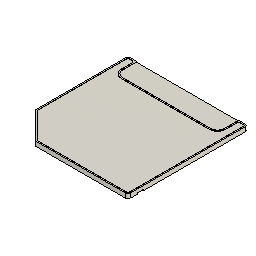
L_Floppy_Disk_v4 (Autodesk Fusion 360 design; units mm, degrees)
Autodesk Fusion 360 part; units mm, degrees
sketch "Sketch1" plane through (0, 0, 0) normal (0, 0, 1) x (1, 0, 0)
  line L0 (-64, 66.5) -> (64, 66.5)
  line L1 (66.5, 64) -> (66.5, -64)
  line L2 (64, -66.5) -> (-36.5, -66.5)
  line L3 (-66.5, -36.5) -> (-66.5, 64)
  line L4 (-36.5, -66.5) -> (-66.5, -36.5)
  arc A0 (-64, 66.5) -> (-66.5, 64) centre (-64, 64) ccw
  arc A1 (66.5, 64) -> (64, 66.5) centre (64, 64) ccw
  arc A2 (64, -66.5) -> (66.5, -64) centre (64, -64) ccw
extrude "Extrude1" add sketch "Sketch1" along normal blind 5
sketch "Sketch2" plane through (0, 0, 5) normal (0, 0, 1) x (-1, 0, 0)
  line L0 (36.5, 66.5) -> (-64, 66.5)
  arc A0 (-64, 66.5) -> (-66.5, 64) centre (-64, 64) ccw
  line L1 (-66.5, 64) -> (-66.5, -64)
  arc A1 (-66.5, -64) -> (-64, -66.5) centre (-64, -64) ccw
  line L2 (-64, -66.5) -> (64, -66.5)
  arc A2 (64, -66.5) -> (66.5, -64) centre (64, -64) ccw
  line L3 (66.5, -64) -> (66.5, 36.5)
  line L4 (66.5, 36.5) -> (36.5, 66.5)
  circle A3 centre (0, 0) radius 20
  circle A4 centre (0, 0) radius 16.5
  line L5 (-56.5, -66.5) -> (56.5, -66.5)
  line L6 (56.5, -66.5) -> (56.5, -50.5727)
  line L7 (49, -43.0727) -> (-49, -43.0727)
  line L8 (-56.5, -50.5727) -> (-56.5, -66.5)
  arc A5 (56.5, -50.5727) -> (49, -43.0727) centre (49, -50.5727) ccw
  arc A6 (-49, -43.0727) -> (-56.5, -50.5727) centre (-49, -50.5727) ccw
  constraint coincident A3.centre A4.centre
  constraint horizontal L5
  constraint equal A5 A6
extrude "Extrude2" cut sketch "Sketch2" against normal blind 0.2 contours L2 L5 L6 L7 L8 A5 A6
extrude "Extrude3" cut 1 faces at (16.3333, 58.6909, 4.8) along direction (0, 0, 1) blind 0.2 from surface at -4.8
sketch "Sketch3" plane through (0, 66.5, 0) normal (0, 1, 0) x (-1, 0, 0)
  line L0 (-56.5, 0) -> (-56.5, 0.2)
  line L1 (-56.5, 0.2) -> (56.5, 0.2)
  line L2 (56.5, 0.2) -> (56.5, 0)
  line L3 (56.5, 0) -> (64, 0)
  line L4 (64, 0) -> (64, 5)
  line L5 (64, 5) -> (56.5, 5)
  line L6 (56.5, 5) -> (56.5, 4.8)
  line L7 (56.5, 4.8) -> (-56.5, 4.8)
  line L8 (-56.5, 4.8) -> (-56.5, 5)
  line L9 (-56.5, 5) -> (-64, 5)
  line L10 (-64, 5) -> (-64, 0)
  line L11 (-64, 0) -> (-56.5, 0)
  line L12 (-56.5, 4.8) -> (56.5, 4.8)
  line L13 (56.5, 4.8) -> (56.5, 0.2)
  line L14 (56.5, 0.2) -> (-56.5, 0.2)
  line L15 (-56.5, 0.2) -> (-56.5, 4.8)
  constraint horizontal L12
  constraint vertical L13
  constraint horizontal L14
  constraint vertical L15
  constraint coincident L1.end L2.start
  constraint coincident L7.end L8.start
extrude "Extrude4" cut sketch "Sketch3" against normal blind 0.2 contours L1 L7 L12 L13 L14 L15
fillet "Fillet1" radius 0.5 2 edges at (0, 66.3, 4.8) (0, 66.3, 0.2)
sketch "Sketch4" plane through (0, 0, 5) normal (0, 0, 1) x (-1, 0, 0)
  line L0 (56.5, -50.5727) -> (56.5, -66.5)
  line L1 (56.5, -66.5) -> (64, -66.5)
  arc A0 (64, -66.5) -> (66.5, -64) centre (64, -64) ccw
  line L2 (66.5, -64) -> (66.5, 36.5)
  line L3 (66.5, 36.5) -> (36.5, 66.5)
  line L4 (36.5, 66.5) -> (-64, 66.5)
  arc A1 (-64, 66.5) -> (-66.5, 64) centre (-64, 64) ccw
  line L5 (-66.5, 64) -> (-66.5, -64)
  arc A2 (-66.5, -64) -> (-64, -66.5) centre (-64, -64) ccw
  line L6 (-64, -66.5) -> (-56.5, -66.5)
  line L7 (-56.5, -66.5) -> (-56.5, -50.5727)
  arc A3 (-49, -43.0727) -> (-56.5, -50.5727) centre (-49, -50.5727) ccw
  line L8 (-49, -43.0727) -> (49, -43.0727)
  arc A4 (56.5, -50.5727) -> (49, -43.0727) centre (49, -50.5727) ccw
  line L9 (-64, 66.5) -> (36.5, 66.5)
  line L10 (66.5, 36.5) -> (66.5, -64)
  line L11 (36.5, 66.5) -> (66.5, 36.5)
  arc A5 (64, -66.5) -> (66.5, -64) centre (64, -64) ccw
  line L12 (-66.5, -64) -> (-66.5, 64)
  arc A6 (-64, 66.5) -> (-66.5, 64) centre (-64, 64) ccw
  arc A7 (-66.5, -64) -> (-64, -66.5) centre (-64, -64) ccw
  line L13 (-56.5, -66.5) -> (-56.5, -50.5727)
  line L14 (-49, -43.0727) -> (49, -43.0727)
  line L15 (56.5, -50.5727) -> (56.5, -66.5)
  arc A8 (56.5, -50.5727) -> (49, -43.0727) centre (49, -50.5727) ccw
  arc A9 (-49, -43.0727) -> (-56.5, -50.5727) centre (-49, -50.5727) ccw
  line L16 (-64, -66.5) -> (-56.5, -66.5)
  line L17 (56.5, -66.5) -> (64, -66.5)
  line L18 (58, -65) -> (64, -65)
  arc A10 (64, -65) -> (65, -64) centre (64, -64) ccw
  line L19 (65, 35.8787) -> (65, -64)
  line L20 (35.8787, 65) -> (65, 35.8787)
  line L21 (-64, 65) -> (35.8787, 65)
  arc A11 (-64, 65) -> (-65, 64) centre (-64, 64) ccw
  line L22 (-65, -64) -> (-65, 64)
  arc A12 (-65, -64) -> (-64, -65) centre (-64, -64) ccw
  line L23 (-64, -65) -> (-58, -65)
  line L24 (-58, -65) -> (-58, -50.5727)
  arc A13 (-49, -41.5727) -> (-58, -50.5727) centre (-49, -50.5727) ccw
  line L25 (-49, -41.5727) -> (49, -41.5727)
  arc A14 (58, -50.5727) -> (49, -41.5727) centre (49, -50.5727) ccw
  line L26 (58, -50.5727) -> (58, -65)
  dimension "d23" = 7.5
  dimension "d24" = -1.5
  constraint vertical L13
  constraint horizontal L14
  constraint vertical L15
  constraint coincident L0.end L1.start
  constraint tangent L14 A8
  constraint tangent L15 A8
  constraint tangent L13 A9
  constraint tangent L14 A9
  constraint equal A8 A9
  constraint coincident A2.end L6.start
  constraint tangent A7 L16
  constraint coincident L1.end A0.start
  constraint tangent A5 L17
  measures "d23" radius of A8
extrude "Extrude5" cut sketch "Sketch4" against normal blind 0.2 contours L18 A10 L19 L20 L21 A11 L22 A12 L23 L24 A13 L25 A14 L26
extrude "Extrude6" cut 1 faces at (25.7071, -29.4758, 4.8) along direction (0, 0, 1) blind 0.2 from surface at -4.8
fillet "Fillet2" radius 2.5 4 edges at (58, 65, 4.9) (-58, 65, 4.9) (-35.8787, -65, 4.9) (-65, -35.8787, 4.9)
extrude "Extrude7" cut sketch "Sketch2" along normal blind 1 from surface at -4.8 contours A3
sketch "Sketch5" plane through (0, 0, 0.2) normal (0, 0, -1) x (1, 0, 0)
  circle A0 centre (0, 0) radius 16.5
  line L0 (2, 0) -> (2, 2)
  line L1 (2, 2) -> (0, 2)
  line L2 (2, 2) -> (-2, 2)
  line L3 (-2, 2) -> (-2, -2)
  line L4 (-2, -2) -> (2, -2)
  line L5 (2, -2) -> (2, 2)
  line L6 (-11, 7) -> (-8, 5)
  line L7 (-8, 5) -> (-4.7692, 9.8462)
  line L8 (-4.7692, 9.8462) -> (-7.7692, 11.8462)
  line L9 (-7.7692, 11.8462) -> (-11, 7)
  constraint vertical L0
  constraint horizontal L1
  constraint horizontal L2
  constraint vertical L3
  constraint horizontal L4
  constraint vertical L5
  constraint perpendicular L6 L7
  constraint parallel L6 L8
  constraint parallel L7 L9
extrude "Extrude8" cut sketch "Sketch5" against normal blind 1 contours L0 L1 L2 L3 L4 L5 | L6 L7 L8 L9
sketch "Sketch6" plane through (0, 0, 0.2) normal (0, 0, -1) x (1, 0, 0)
  arc A0 (-49, -41.5727) -> (-58, -50.5727) centre (-49, -50.5727) ccw
  line L0 (-49, -41.5727) -> (49, -41.5727)
  arc A1 (58, -50.5727) -> (49, -41.5727) centre (49, -50.5727) ccw
  line L1 (58, -50.5727) -> (58, -65)
  line L2 (58, -65) -> (64, -65)
  arc A2 (64, -65) -> (65, -64) centre (64, -64) ccw
  line L3 (65, -64) -> (65, 64)
  arc A3 (65, 64) -> (64, 65) centre (64, 64) ccw
  line L4 (64, 65) -> (-35.8787, 65)
  line L5 (-35.8787, 65) -> (-65, 35.8787)
  line L6 (-65, 35.8787) -> (-65, -64)
  arc A4 (-65, -64) -> (-64, -65) centre (-64, -64) ccw
  line L7 (-64, -65) -> (-58, -65)
  line L8 (-58, -65) -> (-58, -50.5727)
  circle A5 centre (0, 0) radius 20
  line L9 (65, 55.4608) -> (60, 55.4608)
  line L10 (60, 49.4608) -> (65, 49.4608)
  line L11 (65, 49.4608) -> (65, 55.4608)
  arc A6 (60, 55.4608) -> (57, 52.4608) centre (60, 52.4608) ccw
  arc A7 (57, 52.4608) -> (60, 49.4608) centre (60, 52.4608) ccw
  arc A8 (55.5, 52.4608) -> (60, 47.9608) centre (60, 52.4608) ccw
  line L12 (60, 47.9608) -> (66.5, 47.9608)
  line L13 (66.5, 47.9608) -> (66.5, 56.9608)
  line L14 (66.5, 56.9608) -> (60, 56.9608)
  arc A9 (60, 56.9608) -> (55.5, 52.4608) centre (60, 52.4608) ccw
  point P0 (57, 55.4608)
  dimension "d40" = 6
  dimension "d43" = 1.5
  constraint horizontal L9
  constraint horizontal L10
  constraint vertical L11
  constraint coincident L3 L9.start
  constraint coincident P0 L9
  constraint tangent L9 A6
  constraint tangent L10 A7
  constraint coincident A6.end A7.start
  measures "d40" distance of L9.start L10.end
extrude "Extrude9" add sketch "Sketch6" along normal blind 0.2 contours L3 L9 L10 A6 A7 A8 L12 L14 A9
extrude "Extrude10" cut 1 faces at (61.6667, -53.4608, 0.2) along direction (0, 0, 1) blind 1
extrude "Extrude11" cut 1 faces at (65, -53.4608, 0.8) along direction (1, 0, 0) blind 4.5
named bodies: "L_Floppy"
